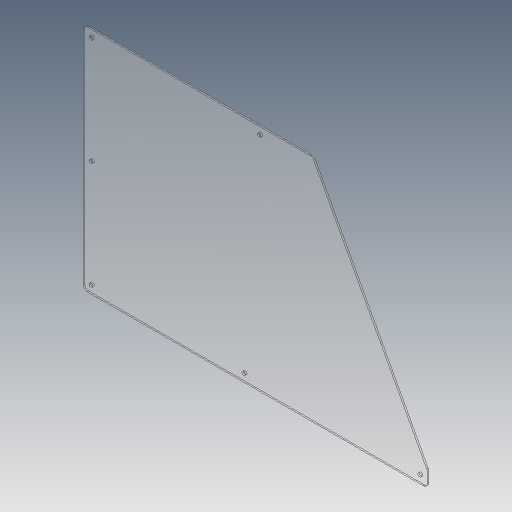
# Autodesk Inventor part: 防水1
Saved by Autodesk Inventor 2020.3 (Build 243373000, 373)
## iProperties
Part Number: 防水1
Material: PET プラスチック
Document SubType Name: Modeling
Designer: highs
Density: 1.541 g/cm^3
Appearance: ポリカーボネート - クリア
Author: highs
Autodesk Inventor part; units mm, degrees
ref_plane "YZ Plane" through (0, 0, 0) normal (1, 0, 0) x (0, 1, 0)
ref_plane "XZ Plane" through (0, 0, 0) normal (0, 1, 0) x (-1, 0, 0)
ref_plane "XY Plane" through (0, 0, 0) normal (0, 0, 1) x (1, 0, 0)
sketch "スケッチ1" plane through (0, 0, 0) normal (0, 0, 1) x (1, 0, 0)
  line L0 (0, 0) -> (450, 0)
  line L1 (450, 0) -> (450, 20)
  line L2 (450, 20) -> (300, 300)
  line L3 (300, 300) -> (0, 300)
  line L4 (0, 300) -> (0, 0)
  line L5 (10, 290) -> (294.0126, 290) construction
  line L6 (294.0126, 290) -> (444.0126, 10) construction
  line L7 (444.0126, 10) -> (10, 10) construction
  line L8 (10, 10) -> (10, 290) construction
  circle A0 centre (10, 290) radius 2.5
  circle A1 centre (10, 10) radius 2.5
  circle A2 centre (10, 150) radius 2.5
  circle A3 centre (210, 10) radius 2.5
  circle A4 centre (440, 10) radius 2.5
  circle A5 centre (230, 290) radius 2.5
  dimension "d0" = 300
  dimension "d1" = 450
  dimension "d2" = 300
  dimension "d3" = 20
  dimension "d6" = 10
  dimension "d7" = 5
  dimension "d8" = 10
  dimension "d9" = 200
  dimension "d10" = 220
  constraints: 18 end point, 6 centre point, 5 equal radius, 3 perpendicular, 3 point on line, 2 coincident, 2 parallel, 1 horizontal, 1 midpoint, 3 other
  measures "d0" distance of L3.end L0.start
  measures "d1" distance of L0.start L0.end
  measures "d2" distance of L2.end L3.end
  measures "d3" distance of L0.end L1.end
  measures "d6" distance between parallel lines of L3 L5
  measures "d7" diameter of A0
  measures "d8" distance from line of L1 A4.centre
  measures "d9" distance from line of L8 A3.centre
  measures "d10" distance of A0.centre A5.centre
extrude "押し出し1" add sketch "スケッチ1" along normal blind 2
fillet "フィレット1" radius 5 5 edges at (450, 0, 1) (450, 20, 1) (0, 0, 1) (300, 300, 1) (0, 300, 1)
